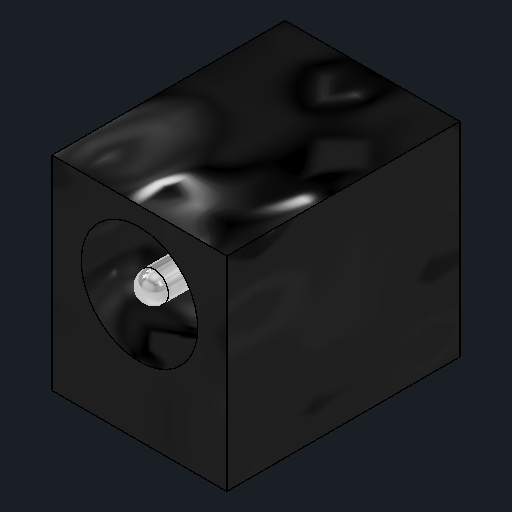
# Autodesk Inventor part: Plug
Saved by Autodesk Inventor 2026.2 (Build 302298000, 298)
## iProperties
Created: 2015-05-06
Part Number: Plug
Material: Generic
Document SubType Name: Modeling
Designer: Philip
Density: 1 g/cm^3
Appearance: Black
Author: Philip
Autodesk Inventor part; units mm, degrees
ref_plane "YZ Plane" through (0, 0, 0) normal (1, 0, 0) x (0, 1, 0)
ref_plane "XZ Plane" through (0, 0, 0) normal (0, 1, 0) x (-1, 0, 0)
ref_plane "XY Plane" through (0, 0, 0) normal (0, 0, 1) x (1, 0, 0)
sketch "Sketch1" plane through (0, 0, 0) normal (0, 0, 1) x (1, 0, 0)
  line L0 (-4.7625, -6.9215) -> (4.7625, -6.9215)
  line L1 (4.7625, -6.9215) -> (4.7625, 4.191)
  line L2 (4.7625, 4.191) -> (-4.7625, 4.191)
  line L3 (-4.7625, 4.191) -> (-4.7625, -6.9215)
  point P0 (0, 0)
  dimension "d0" = 9.525
  dimension "d1" = 11.1125
  dimension "d2" = 4.7625
  dimension "d3" = 4.191
  constraints: 8 end point, 2 parallel, 1 horizontal, 1 perpendicular
  measures "d0" distance of L0.start L0.end
  measures "d1" distance of L0.end L1.end
  measures "d2" distance from line of L1 point (0, 0)
  measures "d3" distance from line of L2 point (0, 0)
extrude "Extrusion1" add sketch "Sketch1" along normal blind 12.7
sketch "Sketch2" plane through (0, 0, 12.7) normal (0, 0, 1) x (1, 0, 0)
  circle A0 centre (0, 0) radius 3.175
  dimension "d6" = 6.35
  constraints: 1 centre point, 1 coincident
  measures "d6" diameter of A0
extrude "Extrusion2" cut sketch "Sketch2" against normal blind 7.62
sketch "Sketch3" plane through (0, 0, 5.08) normal (0, 0, 1) x (1, 0, 0)
  circle A0 centre (0, 0) radius 0.7937
  dimension "d9" = 1.5875
  constraints: 1 centre point, 1 coincident
  measures "d9" diameter of A0
extrude "Extrusion3" add sketch "Sketch3" along normal blind 7.62
fillet "Fillet1" radius 0.7937 1 edges at (-0.7937, 0, 12.7)
equation "\"d2\" = 0.5 * d0"
body "Solid1"
